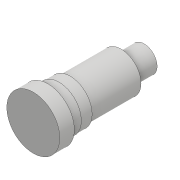
# Autodesk Inventor part: 0871 Spring Loaded
Saved by Autodesk Inventor 2018 (Build 220112000, 112)
## iProperties
Created: 2017-05-10
Part Number: 0871 Spring Loaded
Material: Generic
Document SubType Name: Modeling
Designer: sawaiz
Density: 1 g/cm^3
Appearance: Default
Author: sawaiz
Autodesk Inventor part; units mm, degrees
ref_plane "YZ Plane" through (0, 0, 0) normal (1, 0, 0) x (0, 1, 0)
ref_plane "XZ Plane" through (0, 0, 0) normal (0, 1, 0) x (-1, 0, 0)
ref_plane "XY Plane" through (0, 0, 0) normal (0, 0, 1) x (1, 0, 0)
sketch "Sketch1" plane through (0, 0, 0) normal (0, 0, 1) x (1, 0, 0)
  line L0 (0, 0) -> (-2.375, 0)
  line L1 (-1.97, 2.3) -> (-1.97, 3.3)
  line L2 (-1.97, 3.3) -> (-1.78, 3.3)
  line L3 (-1.78, 3.3) -> (-1.78, 7.87)
  line L4 (-1.78, 7.87) -> (-1.17, 7.87)
  line L5 (-1.17, 7.87) -> (-1.17, 9.9224)
  arc A0 (0, 10.16) -> (-1.17, 9.9224) centre (0, 7.16) ccw
  line L6 (0, 0) -> (0, 10.16)
  line L7 (-1.97, 2.3) -> (-2.005, 2.3)
  line L8 (-2.005, 2.3) -> (-2.005, 1.3)
  line L9 (-2.005, 1.3) -> (-2.375, 1.3)
  line L10 (-2.375, 1.3) -> (-2.375, 0)
  dimension "d0" = 1.17
  dimension "d1" = 1.78
  dimension "d2" = 1.97
  dimension "d3" = 2.005
  dimension "d4" = 2.375
  dimension "d5" = 1.3
  dimension "d6" = 7.87
  dimension "d7" = 2.29
  dimension "d8" = 1
  dimension "d9" = 1
  dimension "d10" = 3
  constraints: 22 end point, 5 perpendicular, 2 horizontal, 2 point on circle, 2 vertical, 1 centre point, 1 line through centre
  measures "d0" distance between parallel lines of L6 L5
  measures "d1" distance between parallel lines of L6 L3
  measures "d2" distance between parallel lines of L6 L1
  measures "d3" distance between parallel lines of L6 L8
  measures "d4" distance between parallel lines of L6 L10
  measures "d5" distance of L9.end L0.end
  measures "d6" distance between parallel lines of L0 L4
  measures "d7" vertical distance of L3.end L6.end
  measures "d8" distance of L7.end L8.end
  measures "d9" distance between parallel lines of L7 L2
  measures "d10" radius of A0
revolve "Revolution1" add sketch "Sketch1" angle 360 about axis through (0, 0, 0) along (0, 1, 0)
body "Solid1"
